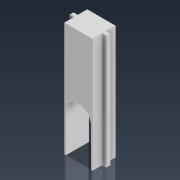
# Autodesk Inventor part: Slider-6
Saved by Autodesk Inventor 2021.1 (Build 251245010, 245A)
## iProperties
Created: 2020-12-20
Part Number: Slider-6
Material: 一般
Document SubType Name: Modeling
Designer: User
Density: 1 g/cm^3
Appearance: 預設
Author: User
Autodesk Inventor part; units mm, degrees
ref_plane "YZ Plane" through (0, 0, 0) normal (1, 0, 0) x (0, 1, 0)
ref_plane "XZ Plane" through (0, 0, 0) normal (0, 1, 0) x (-1, 0, 0)
ref_plane "XY Plane" through (0, 0, 0) normal (0, 0, 1) x (1, 0, 0)
sketch "草圖1" plane through (0, 0, 0) normal (0, 1, 0) x (-1, 0, 0)
  line L0 (-33.5, 27) -> (33.5, 27)
  line L1 (33.5, 27) -> (33.5, -27)
  line L2 (33.5, -27) -> (-33.5, -27)
  line L3 (-33.5, -27) -> (-33.5, 27)
  line L4 (-33.5, 27) -> (33.5, -27) construction
  line L5 (33.5, 27) -> (-33.5, -27) construction
  line L6 (43.5, -4.5) -> (33.5, -4.5)
  line L7 (33.5, -4.5) -> (33.5, 4.5)
  line L8 (33.5, 4.5) -> (43.5, 4.5)
  line L9 (43.5, 4.5) -> (43.5, -4.5)
  line L10 (-33.5, -4.5) -> (-43.5, -4.5)
  line L11 (-43.5, -4.5) -> (-43.5, 4.5)
  line L12 (-43.5, 4.5) -> (-33.5, 4.5)
  line L13 (-33.5, 4.5) -> (-33.5, -4.5)
  point P0 (0, 0)
  point P1 (33.5, 0)
  point P2 (-33.5, 0)
  point P3 (-33.5, 4.5)
  point P4 (-33.5, -4.5)
  dimension "d0" = 67
  dimension "d1" = 54
  dimension "d2" = 9
  dimension "d3" = 10
  constraints: 28 end point, 6 midpoint, 6 parallel, 3 horizontal, 3 perpendicular, 2 equal length
  measures "d0" distance of L0.start L0.end
  measures "d1" distance of L2.end L0.start
  measures "d2" distance of L8.end L6.start
  measures "d3" distance of L6.start L6.end
extrude "擠出1" add sketch "草圖1" along normal blind 350
sketch "草圖2" plane through (-33.5, 0, 27) normal (0, 0, 1) x (1, 0, 0)
  line L0 (0, 0) -> (0, 350) projected
  line L1 (0, 350) -> (67, 350) projected
  line L2 (67, 350) -> (67, 0) projected
  line L3 (67, 0) -> (0, 0) projected
  circle A0 centre (33.5, 148) radius 30
  line L4 (3.5, 148) -> (63.5, 148)
  line L5 (63.5, 148) -> (63.5, -3.654)
  line L6 (63.5, -3.654) -> (3.5, -3.654)
  line L7 (3.5, -3.654) -> (3.5, 148)
  point P0 (33.5, 0)
  point P1 (33.5, 0)
  point P2 (63.5, 148)
  point P3 (3.5, 148)
  dimension "d6" = 148
  dimension "d7" = 60
  constraints: 8 end point, 2 midpoint, 2 parallel, 1 centre point, 1 coincident, 1 horizontal, 1 perpendicular, 1 tangent, 1 vertical alignment
  measures "d6" distance from line of L3 A0.centre
  measures "d7" diameter of A0
extrude "擠出2" cut sketch "草圖2" against normal through all contours L7 A0 L5 L3 | L3 L5 L6 L7 | L4 A0 | A0 L4
sketch "草圖3" plane through (-33.5, 350, 27) normal (0, 0, 1) x (1, 0, 0)
  line L0 (-135.2961, -270) -> (202.2961, -270)
  line L1 (202.2961, -270) -> (202.2961, -350)
  line L2 (202.2961, -350) -> (-135.2961, -350)
  line L3 (-135.2961, -350) -> (-135.2961, -270)
  point P0 (33.5, -350)
  point P1 (33.5, -350)
  dimension "d10" = 80
  constraints: 8 end point, 2 parallel, 1 coincident, 1 horizontal, 1 midpoint, 1 perpendicular
  measures "d10" distance of L0.end L1.end
extrude "擠出3" cut sketch "草圖3" against normal through all
sketch "草圖4" plane through (33.5, 350, -27) normal (0, 0, -1) x (-1, 0, 0)
  arc A0 (63.5, -202) -> (3.5, -202) centre (33.5, -202) ccw construction
  circle A1 centre (33.5, -182) radius 30
  line L0 (63.5, -270) -> (3.5, -270)
  line L1 (3.5, -270) -> (3.5, -182)
  line L2 (3.5, -182) -> (63.5, -182)
  line L3 (63.5, -182) -> (63.5, -270)
  line L4 (63.5, -270) -> (67, -270) projected
  point P0 (33.5, -350)
  point P1 (65.25, -270)
  dimension "d13" = 20
  dimension "d14" = 60
  constraints: 8 end point, 2 midpoint, 2 parallel, 1 centre point, 1 coincident, 1 horizontal, 1 horizontal alignment, 1 perpendicular, 1 tangent, 1 vertical alignment
  measures "d13" distance of A0.centre A1.centre
  measures "d14" diameter of A1
sketch "草圖5" plane through (-33.5, 350, 27) normal (0, 0, 1) x (1, 0, 0)
  arc A0 (63.5, -202) -> (3.5, -202) centre (33.5, -202) ccw construction
  circle A1 centre (33.5, -180) radius 30
  line L0 (63.5, -270) -> (3.5, -270)
  line L1 (3.5, -270) -> (3.5, -180)
  line L2 (3.5, -180) -> (63.5, -180)
  line L3 (63.5, -180) -> (63.5, -270)
  point P0 (33.5, -350)
  point P1 (63.5, -270)
  dimension "d15" = 22
  dimension "d16" = 60
  constraints: 8 end point, 2 coincident, 2 parallel, 1 centre point, 1 horizontal, 1 midpoint, 1 perpendicular, 1 tangent, 1 vertical alignment
  measures "d15" distance of A0.centre A1.centre
  measures "d16" diameter of A1
loft "斷面混成1" cut profiles "草圖4", "草圖5"
